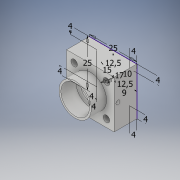
# Autodesk Inventor part: Oberteil_Zerstäuber
Saved by Autodesk Inventor 2019 (Build 230136000, 136)
## iProperties
Created: 2018-09-03
Part Number: Oberteil_Zerstäuber
Material: Generisch
Document SubType Name: Modeling
Designer: kenoe
Density: 1 g/cm^3
Appearance: Vorgabe
Author: kenoe
Autodesk Inventor part; units mm, degrees
ref_plane "YZ Plane" through (0, 0, 0) normal (1, 0, 0) x (0, 1, 0)
ref_plane "XZ Plane" through (0, 0, 0) normal (0, 1, 0) x (-1, 0, 0)
ref_plane "XY Plane" through (0, 0, 0) normal (0, 0, 1) x (1, 0, 0)
sketch "Skizze1" plane through (0, 0, 0) normal (0, 0, 1) x (1, 0, 0)
  line L0 (12.5, -12.5) -> (-12.5, -12.5)
  line L1 (-12.5, -12.5) -> (-12.5, 12.5)
  line L2 (-12.5, 12.5) -> (12.5, 12.5)
  line L3 (12.5, 12.5) -> (12.5, -12.5)
  circle A0 centre (0, 0) radius 5
  circle A1 centre (0, 0) radius 7.5
  circle A2 centre (0, 0) radius 8.5
  circle A3 centre (0, 0) radius 4.5
  point P0 (-8.5, 8.5)
  point P1 (8.5, 8.5)
  point P2 (8.5, -8.5)
  point P3 (-8.5, -8.5)
  dimension "d0" = 25
  dimension "d1" = 25
  dimension "d2" = 4
  dimension "d3" = 4
  dimension "d4" = 4
  dimension "d5" = 4
  dimension "d6" = 10
  dimension "d7" = 15
  dimension "d8" = 17
  dimension "d11" = 9
  dimension "d18" = 12.5
  dimension "d19" = 12.5
  dimension "d21" = 4
  dimension "d38" = 4
  dimension "d39" = 4
  dimension "d48" = 4
  constraints: 8 end point, 4 centre point, 4 coincident, 2 parallel, 1 horizontal, 1 perpendicular
  measures "d0" distance of L1.end L2.end
  measures "d1" distance of L0.end L1.end
  measures "d2" distance from line of L2 point (8.5, 8.5)
  measures "d3" distance from line of L3 point (8.5, -8.5)
  measures "d4" distance from line of L0 point (-8.5, -8.5)
  measures "d5" distance from line of L1 point (-8.5, 8.5)
  measures "d6" diameter of A0
  measures "d7" diameter of A1
  measures "d8" diameter of A2
  measures "d11" diameter of A3
  measures "d18" distance from line of point (0, 0) L3
  measures "d19" distance from line of point (0, 0) L2
  measures "d21" distance from line of point (8.5, 8.5) L3
  measures "d38" distance from line of L1 point (-8.5, -8.5)
  measures "d39" distance from line of L2 point (-8.5, 8.5)
  measures "d48" distance from line of L0 point (8.5, -8.5)
sketch "Skizze2" plane through (0, 0, 0) normal (1, 0, 0) x (0, 1, 0)
  line L0 (0, 0) -> (0, 10)
  dimension "d47" = 10
  constraints: 2 end point, 1 coincident, 1 vertical
  measures "d47" distance of L0.start L0.end
extrude "Extrusion2" add sketch "Skizze1" along normal blind 20 contours A2
extrude "Extrusion3" add sketch "Skizze1" along normal blind 12 separate body contours L0 L1 L2 L3 | A1
extrude "Extrusion4" add sketch "Skizze1" along normal blind 6.4 separate body contours A0
hole "Bohrung2" at (8.5, -8.5, 0) at (8.5, 8.5, 0) at (-8.5, 8.5, 0) at (-8.5, -8.5, 0) direction (0, 0, 1) diameter 3.4 end through all counterbore diameter 6.5 counterbore depth 3.4 bodies 2 clearance for "Inbusschraube DIN EN ISO 4762" size "M3" standard "DIN"
hole "Bohrung3" at (0, 0, 10) direction (1, 0, 0) diameter 2.057 end through all bodies 2
